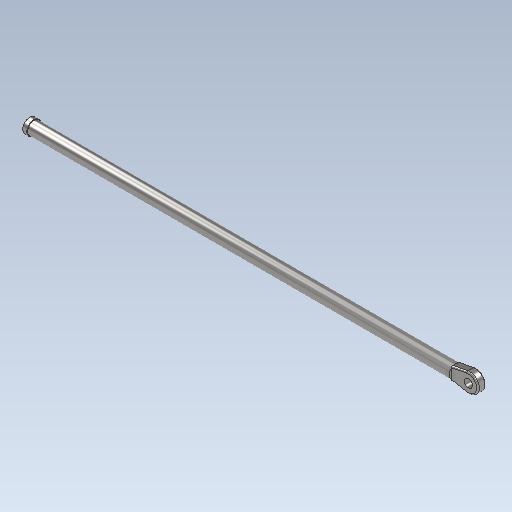
# Autodesk Inventor part: Lift.02.00.00.05
Saved by Autodesk Inventor 2021 (Build 250183000, 183)
## iProperties
Created: 2020-09-20
Part Number: Lift.02.00.00.05
Material: Сталь нержавеющая, 440C
Document SubType Name: Modeling
Designer: Kostya
Density: 7.75 g/cm^3
Appearance: С умеренной полировкой
Author: Kostya
Autodesk Inventor part; units mm, degrees
ref_plane "YZ Plane" through (0, 0, 0) normal (1, 0, 0) x (0, 1, 0)
ref_plane "XZ Plane" through (0, 0, 0) normal (0, 1, 0) x (-1, 0, 0)
ref_plane "XY Plane" through (0, 0, 0) normal (0, 0, 1) x (1, 0, 0)
sketch "Эскиз1" plane through (0, 0, 0) normal (0, 0, 1) x (1, 0, 0)
  line L0 (0, 0) -> (-3498.9825, 0)
  line L1 (0, 0) -> (0, 72.2666) construction
  line L2 (0, 47.5) -> (-3077, 47.5)
  line L3 (-3077, 47.5) -> (-3077, 52.5)
  line L4 (-3077, 52.5) -> (-3107, 52.5)
  line L5 (-3107, 52.5) -> (-3107, 0)
  line L6 (0, 0) -> (0, 47.5)
  point P0 (-3107, 0)
  dimension "d1" = 105
  dimension "d2" = 95
  dimension "d3" = 30
  dimension "d4" = 3107
  constraints: 14 end point, 3 perpendicular, 2 horizontal, 1 collinear, 1 point on line, 1 vertical
  measures "d1" diameter of L4 L0
  measures "d2" diameter of L2 L0
  measures "d3" distance of L3.end L4.end
  measures "d4" distance from line of L2.start L5
revolve "Вращение1" add sketch "Эскиз1" angle 360 about axis through (0, 0, 0) along (-1, 0, 0)
sketch "Эскиз2" plane through (0, 0, 0) normal (0, 0, 1) x (1, 0, 0)
  line L0 (-3077, -47.5) -> (-3077, 47.5) projected
  line L1 (0, -47.5) -> (0, 47.5) projected
  circle A0 centre (123.2661, 0) radius 30
  circle A1 centre (123.2661, 0) radius 70
  line L2 (110, -68.7314) -> (0, -47.5)
  line L3 (0, -47.5) -> (0, 47.5) projected
  line L4 (0, 47.5) -> (110, 68.7314)
  point P0 (0, 0)
  point P1 (0, 0)
  dimension "d6" = 60
  dimension "d7" = 140
  dimension "d8" = 110
  constraints: 4 end point, 2 centre point, 2 point on circle, 2 tangent, 1 coincident, 1 horizontal alignment, 1 midpoint
  measures "d6" diameter of A0
  measures "d7" diameter of A1
  measures "d8" horizontal distance of L2.start L1.start
extrude "Выдавливание1" add sketch "Эскиз2" along normal mid plane 60
fillet "Сопряжение1" radius 10 6 edges at (193.2661, 0, 30) (55, -58.1157, 30) (55, 58.1157, 30) (55, -58.1157, -30) (55, 58.1157, -30) (193.2661, 0, -30)
